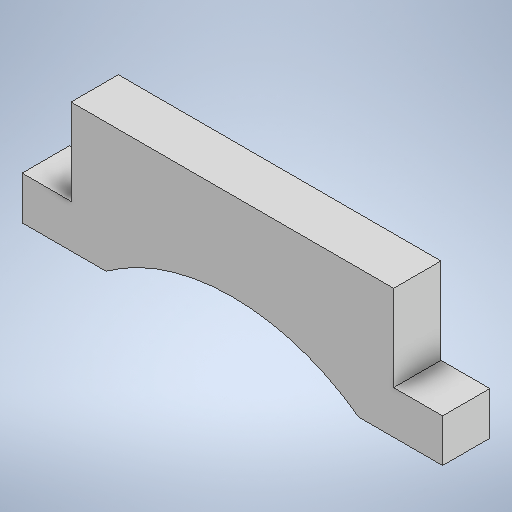
# Autodesk Inventor part: Light Pipe modern
Saved by Autodesk Inventor 2025 (Build 290162000, 162)
## iProperties
Created: 2024-07-18
Part Number: Light Pipe modern
Material: Generic
Document SubType Name: Modeling
Designer: adam
Density: 1 g/cm^3
Appearance: Default
Author: adam
Autodesk Inventor part; units mm, degrees
ref_plane "YZ Plane" through (0, 0, 0) normal (1, 0, 0) x (0, 1, 0)
ref_plane "XZ Plane" through (0, 0, 0) normal (0, 1, 0) x (-1, 0, 0)
ref_plane "XY Plane" through (0, 0, 0) normal (0, 0, 1) x (1, 0, 0)
sketch "Sketch1" plane through (0, 0, 0) normal (0, 0, 1) x (1, 0, 0)
  line L0 (0, 0) -> (15.75, 0)
  line L1 (15.75, 0) -> (15.75, -4)
  line L2 (0, -4) -> (0, 0)
  line L3 (17.65, -4) -> (17.65, -6)
  line L4 (-1.9, -6) -> (-1.9, -4)
  line L5 (-1.9, -4) -> (0, -4)
  line L6 (15.75, -4) -> (17.65, -4)
  line L7 (2, 0) -> (2, -6) construction
  line L8 (13.75, 0) -> (13.75, -6) construction
  arc A0 (13.75, -6) -> (2, -6) centre (7.875, -14.0922) ccw
  line L9 (17.65, -6) -> (13.75, -6)
  line L10 (2, -6) -> (-1.9, -6)
  dimension "d2" = 1.9
  dimension "d3" = 4
  dimension "d4" = 2
  dimension "d5" = 15.75
  dimension "d6" = 2
  dimension "d7" = 2
  dimension "d8" = 10
  constraints: 22 end point, 7 perpendicular, 6 parallel, 3 collinear, 3 horizontal, 2 point on circle, 2 point on line, 1 centre point
  measures "d2" distance of L1.end L3.start
  measures "d3" distance of L2.start L0.start
  measures "d4" distance of L4.start L4.end
  measures "d5" distance of L0.start L0.end
  measures "d6" distance between parallel lines of L7 L2
  measures "d7" distance between parallel lines of L1 L8
  measures "d8" radius of A0
extrude "Extrusion1" add sketch "Sketch1" along normal blind 2.2
sketch "Sketch2" plane through (0, 0, 2.2) normal (0, 0, 1) x (1, 0, 0)
  line L0 (0, 0) -> (0.375, 0)
  line L1 (0.375, 0) -> (0.375, -4)
  line L2 (0.375, -4) -> (0, -4)
  line L3 (0, -4) -> (0, 0)
  line L4 (15.75, 0) -> (0, 0) projected
  line L5 (15.75, 0) -> (15.375, 0)
  line L6 (15.375, 0) -> (15.375, -4)
  line L7 (15.375, -4) -> (15.75, -4)
  line L8 (15.75, -4) -> (15.75, 0)
  dimension "d11" = 15
  dimension "d12" = 4
  constraints: 16 end point, 4 parallel, 2 equal length, 2 horizontal, 2 perpendicular
  measures "d11" distance between parallel lines of L6 L1
  measures "d12" distance of L0.end L1.end
extrude "Extrusion2" cut sketch "Sketch2" against normal up to surface (2.2 mm away)
body "Solid1"
